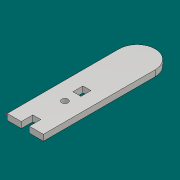
# Autodesk Inventor part: gpu_support
Saved by Autodesk Inventor 2018.2 (Build 222227000, 227)
## iProperties
Created: 2020-08-09
Part Number: gpu_support
Material: アルミニウム 6061
Document SubType Name: Modeling
Designer: gisen
Density: 2.7 g/cm^3
Appearance: アルミニウム - フラット
Author: gisen
Autodesk Inventor part; units mm, degrees
ref_plane "YZ Plane" through (0, 0, 0) normal (1, 0, 0) x (0, 1, 0)
ref_plane "XZ Plane" through (0, 0, 0) normal (0, 1, 0) x (-1, 0, 0)
ref_plane "XY Plane" through (0, 0, 0) normal (0, 0, 1) x (1, 0, 0)
sketch "スケッチ1" plane through (0, 0, 0) normal (0, 0, 1) x (1, 0, 0)
  line L0 (0, 0) -> (7, 0)
  line L1 (7, 0) -> (7, 6)
  line L2 (7, 6) -> (11, 6)
  line L3 (11, 6) -> (11, 0)
  line L4 (11, 0) -> (18, 0)
  line L5 (18, 0) -> (18, 56)
  arc A0 (18, 56) -> (0, 56) centre (9, 56) ccw
  line L6 (0, 0) -> (0, 56)
  line L7 (18, 56) -> (0, 56) construction
  line L8 (9, 6) -> (9, 20) construction
  circle A1 centre (9, 20) radius 1.6
  line L9 (7, 26) -> (11, 26)
  line L10 (11, 26) -> (11, 31)
  line L11 (11, 31) -> (7, 31)
  line L12 (7, 31) -> (7, 26)
  line L13 (9, 56) -> (9, 65) construction
  dimension "d0" = 4
  dimension "d1" = 6
  dimension "d2" = 18
  dimension "d3" = 20
  dimension "d4" = 3.2
  dimension "d5" = 26
  dimension "d6" = 5
  dimension "d7" = 65
  constraints: 28 end point, 5 perpendicular, 4 point on line, 3 horizontal, 3 point on circle, 2 centre point, 2 coincident, 2 midpoint, 2 parallel, 1 collinear, 1 tangent, 1 vertical
  measures "d0" distance of L1.end L2.end
  measures "d1" distance of L2.end L3.end
  measures "d2" distance between parallel lines of L5 L6
  measures "d3" distance from line of L4 L8.end
  measures "d4" diameter of A1
  measures "d5" distance between parallel lines of L4 L9
  measures "d6" distance of L9.end L10.end
  measures "d7" vertical distance of L0.start L13.end
extrude "押し出し1" add sketch "スケッチ1" along normal blind 3
sketch "スケッチ2" plane through (0, 0, 3) normal (0, 0, 1) x (1, 0, 0)
  point P0 (0, 0)
sketch "スケッチ3" plane through (0, 0, 3) normal (0, 0, 1) x (1, 0, 0)
  line L0 (0, 0) -> (7, 0) projected
  line L1 (0, 0) -> (7, 0)
  line L2 (7, 0) -> (7, 0.25)
  line L3 (7, 0.25) -> (0, 0.25)
  line L4 (0, 0.25) -> (0, 0)
  line L5 (11, 0) -> (18, 0) projected
  line L6 (11, 6) -> (11, 0) projected
  line L7 (18, 0) -> (11, 0)
  line L8 (11, 0) -> (11, 0.25)
  line L9 (11, 0.25) -> (18, 0.25)
  line L10 (18, 0.25) -> (18, 0)
  line L11 (7, 0) -> (7, 6) projected
  dimension "d10" = 0.25
  dimension "d11" = 0.25
  constraints: 16 end point, 4 parallel, 2 horizontal, 2 perpendicular, 2 point on line
  measures "d10" distance between parallel lines of L0 L3
  measures "d11" distance between parallel lines of L5 L9
extrude "押し出し2" cut sketch "スケッチ3" against normal through all
equation "\"d11\" = d10"
